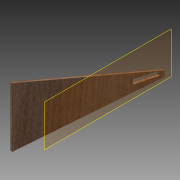
# Autodesk Inventor part: Stand
Saved by Autodesk Inventor 2017 (Build 210142000, 142)
## iProperties
Created: 2018-10-12
Part Number: Stand
Material: Wood (Birch)
Document SubType Name: Modeling
Designer: ari
Density: 0.55 g/cm^3
Appearance: Birch - Natural Polished
Author: ari
Autodesk Inventor part; units mm, degrees
ref_plane "XZ Plane" through (0, 0, 0) normal (0, 1, 0) x (-1, 0, 0)
ref_plane "XY Plane" through (0, 0, 0) normal (0, 0, 1) x (1, 0, 0)
sketch "Sketch1" plane through (0, 0, 0) normal (0, 0, 1) x (1, 0, 0)
  line L0 (-102.7278, -80.4997) -> (-34.2315, 155.1415)
  line L1 (-34.2315, 155.1415) -> (-39.0327, 156.5371)
  line L2 (-39.0327, 156.5371) -> (-107.529, -79.104)
  line L3 (-107.529, -79.104) -> (-102.7278, -80.4997)
  line L4 (-41.9395, 146.5371) -> (-41.9395, 156.5371) construction
  line L5 (-41.9395, 156.5371) -> (-39.0327, 156.5371) construction
  line L6 (-232.529, -80.4997) -> (-232.529, 130.1415) construction
  line L7 (-41.9395, 104.1062) -> (-418.1395, 104.1062) construction
  line L8 (-41.9395, 104.1062) -> (-41.9395, 339.3062) construction
  line L9 (-70.779, -80.4997) -> (-394.279, -80.4997) construction
  dimension "d0" = 5
  dimension "d2" = 10
  dimension "d3" = 125
  constraints: 14 end point, 2 parallel, 2 perpendicular, 1 point on line, 1 vertical
  measures "d0" distance of L2.end L0.start
  measures "d2" distance of L4.start L4.end
  measures "d3" distance from line of L6 L2.end
extrude "Extrusion1" add sketch "Sketch1" against normal blind 5
sketch "Sketch2" plane through (0, 0, 0) normal (0, 0, 1) x (1, 0, 0)
  line L0 (-102.7278, -80.4997) -> (-34.2315, 155.1415) projected
  line L1 (-34.2315, 155.1415) -> (-39.0327, 156.5371) projected
  line L2 (-39.0327, 156.5371) -> (-107.529, -79.104) projected
  line L3 (-107.529, -79.104) -> (-102.7278, -80.4997) projected
  point P0 (0, 0)
ref_plane "Work Plane1" through (-399.029, 141.4738, 12.2861) normal (0, -0.258819, -0.9659258) x (1, 0, 0)
extrude "Extrusion2" add sketch "Sketch2" along normal up to surface surface through (-399.029, 141.4738, 12.2861) normal (0, -0.258819, -0.9659258)
ref_plane "Work Plane2" through (-34.2315, 155.1415, 8.6239) normal (1, 0, 0) x (0, 1, 0)
sketch "Sketch7" plane through (0, 0, 0) normal (0, 0, 1) x (1, 0, 0)
  line L0 (-102.7278, -80.4997) -> (-34.2315, 155.1415) construction
  line L1 (-107.529, -79.104) -> (-39.0327, 156.5371) projected
  line L2 (-39.0327, 156.5371) -> (-34.2315, 155.1415)
  line L3 (-34.2315, 155.1415) -> (-47.3441, 110.0314)
  line L4 (-47.3441, 110.0314) -> (-52.1454, 111.4271)
  line L5 (-52.1454, 111.4271) -> (-39.0327, 156.5371)
  point P0 (0, 0)
  dimension "d19" = 46.9772
  constraints: 8 end point, 2 parallel, 2 perpendicular
  measures "d19" distance between parallel lines of L2 L4
extrude "Extrusion7" add sketch "Sketch7" along normal blind 15
sketch "Sketch3" plane through (-34.2315, 155.1415, 8.6239) normal (1, 0, 0) x (0, 1, 0)
  line L0 (-8.6044, -8.6239) -> (-51.0353, -8.6239) construction
  line L1 (-51.0353, -8.6239) -> (-51.0353, -0.0239) construction
  line L2 (-51.0353, -0.0239) -> (-8.6044, -0.0239) construction
  line L3 (-8.6044, -0.0239) -> (-8.6044, -8.6239) construction
  line L4 (-8.6044, -0.0239) -> (-51.0353, -8.6239) construction
  line L5 (-51.4353, 0.3761) -> (-8.2044, 0.3761)
  line L6 (-8.2044, 0.3761) -> (-8.2044, -9.0239)
  line L7 (-8.2044, -9.0239) -> (-51.4353, -9.0239)
  line L8 (-51.4353, -9.0239) -> (-51.4353, 0.3761)
  line L9 (-51.4353, 0.3761) -> (-8.2044, -9.0239) construction
  line L10 (-8.2044, 0.3761) -> (-51.4353, -9.0239) construction
  line L11 (-51.0353, -0.0239) -> (-51.0353, -8.5239) construction
  point P0 (-155.1415, -8.6239)
  point P1 (-29.8198, -4.3239)
  dimension "d10" = 0.4
  dimension "d11" = 0.4
  constraints: 22 end point, 4 parallel, 3 midpoint, 2 horizontal, 2 perpendicular
  measures "d10" distance between parallel lines of L7 L0
  measures "d11" distance between parallel lines of L6 L3
extrude "Extrusion3" cut sketch "Sketch3" along normal through all both and the other way through all
sketch "Sketch6" plane through (-102.7278, -80.4997, 71.7637) normal (0.9602541, -0.2791272, 0) x (0, 0, -1)
  line L0 (120.0334, 0) -> (76.7637, 0)
  line L1 (76.7637, 245.3946) -> (76.7637, 0) construction
  line L2 (120.0334, 0) -> (76.7637, 245.3946)
  line L3 (76.7637, 245.3946) -> (76.7637, 0)
  dimension "d16" = 10
  constraints: 6 end point, 1 collinear, 1 perpendicular
  measures "d16" angle of L2 L1
extrude "Extrusion6" add sketch "Sketch6" against normal up to surface (5 mm away)
sketch "Sketch8" plane through (-107.529, -79.104, -48.2697) normal (-0.9602541, 0.2791272, 0) x (0, 0, 1)
  line L0 (43.2697, 245.3946) -> (63.2697, 245.3946) projected
  line L1 (0, 0) -> (119.6595, 0) projected
  line L2 (63.2697, 219.1602) -> (119.6595, 0) projected
  line L3 (63.2697, 245.3946) -> (63.2697, 219.1602) projected
  line L4 (57.2697, 235.3972) -> (57.2697, 190.377) projected
  line L5 (57.2697, 190.377) -> (47.8697, 190.377) projected
  line L6 (47.8697, 190.377) -> (47.8697, 235.3972) projected
  line L7 (47.8697, 235.3972) -> (57.2697, 235.3972) projected
  line L8 (0, 0) -> (43.2697, 245.3946) projected
  point P0 (48.2697, 105.9743)
fillet "Fillet1" radius 2 2 edges at (-36.6321, 155.8393, -5) (-36.6321, 155.8393, 15)
fillet "Fillet1" radius 20 1 edges at (-43.752, 131.3455, 15)
body "Solid1"
